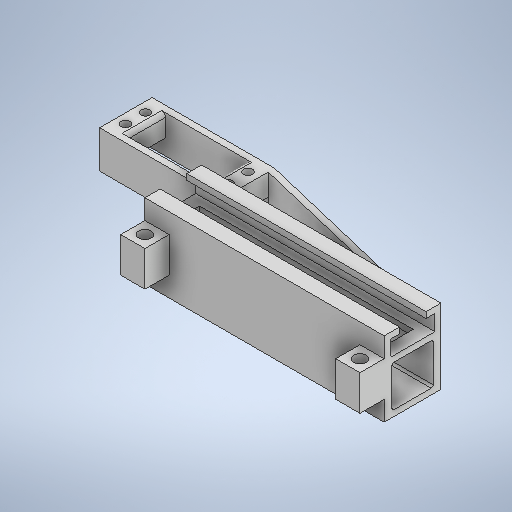
# Autodesk Inventor part: shaftHolder4V1
Saved by Autodesk Inventor 2025.2 (Build 292293000, 293)
## iProperties
Created: 2025-04-03
Part Number: shaftHolder4V1
Material: Generic
Document SubType Name: Modeling
Designer: patrickandersen
Density: 1 g/cm^3
Appearance: Default
Author: patrickandersen
Autodesk Inventor part; units mm, degrees
ref_plane "YZ Plane" through (0, 0, 0) normal (1, 0, 0) x (0, 1, 0)
ref_plane "XZ Plane" through (0, 0, 0) normal (0, 1, 0) x (-1, 0, 0)
ref_plane "XY Plane" through (0, 0, 0) normal (0, 0, 1) x (1, 0, 0)
sketch "Sketch1" plane through (0, 0, 0) normal (0, 1, 0) x (-1, 0, 0)
  line L0 (200.4562, 91.842) -> (79.4562, 91.842)
  line L1 (79.4562, 91.842) -> (79.4562, 63.142)
  line L2 (79.4562, 63.142) -> (200.4562, 63.142)
  line L3 (200.4562, 63.142) -> (200.4562, 91.842)
  point P0 (0, 0)
  dimension "d0" = 121
  dimension "d1" = 28.7
  constraints: 8 end point, 2 parallel, 1 horizontal, 1 perpendicular
  measures "d0" distance of L1.end L2.end
  measures "d1" distance of L0.end L1.end
extrude "Extrusion1" add sketch "Sketch1" along normal blind 26.8
sketch "Sketch2" plane through (-79.4562, 0, 91.842) normal (1, 0, 0) x (0, 0, -1)
  line L0 (4.95, 3) -> (23.75, 3)
  line L1 (24.75, 4) -> (24.75, 22.8)
  line L2 (23.75, 23.8) -> (4.95, 23.8)
  line L3 (3.95, 22.8) -> (3.95, 4)
  line L4 (28.7, 0) -> (28.7, 26.8) projected
  line L5 (0, 0) -> (0, 26.8) projected
  line L6 (0, 26.8) -> (28.7, 26.8) projected
  arc A0 (24.75, 22.8) -> (23.75, 23.8) centre (23.75, 22.8) ccw
  arc A1 (23.75, 3) -> (24.75, 4) centre (23.75, 4) ccw
  arc A2 (3.95, 4) -> (4.95, 3) centre (4.95, 4) ccw
  arc A3 (4.95, 23.8) -> (3.95, 22.8) centre (4.95, 22.8) ccw
  line L7 (0, 0) -> (28.7, 0) projected
  point P0 (91.842, 0)
  point P1 (3.95, 3)
  point P2 (24.75, 23.8)
  point P3 (3.95, 23.8)
  dimension "d4" = 20.8
  dimension "d5" = 20.8
  dimension "d7" = 3.95
  dimension "d8" = 3
  dimension "d9" = 1
  dimension "d137" = 3.95
  dimension "d138" = 3
  constraints: 8 end point, 8 point on circle, 8 tangent, 6 point on line, 4 centre point, 3 equal radius, 2 parallel, 1 horizontal, 1 perpendicular
  measures "d4" distance of point (3.95, 23.8) point (3.95, 3)
  measures "d5" distance of point (24.75, 23.8) point (3.95, 23.8)
  measures "d7" distance between parallel lines of L5 L3
  measures "d8" distance between parallel lines of L6 L2
  measures "d9" radius of A0
  measures "d137" distance between parallel lines of L4 L1
  measures "d138" distance between parallel lines of L7 L0
extrude "Extrusion2" cut sketch "Sketch2" against normal blind 121 contours A2 L3 A3 L2 A0 L1 A1 L0
sketch "Sketch3" plane through (0, 0, 0) normal (0, -1, 0) x (1, 0, 0)
  line L0 (-200.4562, 63.142) -> (-200.4562, 91.842) projected
  line L1 (-200.4562, 91.842) -> (-79.4562, 91.842) projected
  line L2 (-79.4562, 63.142) -> (-200.4562, 63.142) projected
  circle A0 centre (-188.2062, 77.492) radius 9.25
  line L3 (-79.4562, 91.842) -> (-79.4562, 63.142) projected
  point P0 (0, 0)
  dimension "d20" = 14.35
  dimension "d21" = 18.5
  dimension "d287" = 12.25
  constraints: 1 centre point
  measures "d20" distance from line of L1 A0.centre
  measures "d21" diameter of A0
  measures "d287" distance from line of L0 A0.centre
hole "Hole1" at (-188.2062, 0, 77.492) direction (0, 1, 0) diameter 18.5 depth 5
sketch "Sketch4" plane through (0, 26.8, 0) normal (0, 1, 0) x (1, 0, 0)
  line L0 (-85.9562, -84.142) -> (-193.9562, -84.142)
  line L1 (-193.9562, -84.142) -> (-193.9562, -70.642)
  line L2 (-193.9562, -70.642) -> (-85.9562, -70.642)
  line L3 (-85.9562, -70.642) -> (-85.9562, -84.142)
  line L4 (-79.4562, -91.842) -> (-79.4562, -63.142) projected
  line L5 (-200.4562, -63.142) -> (-200.4562, -91.842) projected
  point P0 (0, 0)
  point P1 (-79.4562, -86.142)
  point P2 (-79.4562, -65.142)
  point P3 (-179.4562, -65.142)
  point P4 (-179.4562, -86.142)
  point P5 (-200.4562, -91.842)
  point P6 (-79.4562, -87.892)
  dimension "d30" = 6.5
  dimension "d31" = 6.5
  dimension "d32" = 13.5
  dimension "d41" = 3.75
  constraints: 8 end point, 2 parallel, 1 horizontal, 1 perpendicular, 1 other
  measures "d30" distance between parallel lines of L4 L3
  measures "d32" distance between parallel lines of L0 L2
  measures "d41" distance from line of point (-79.456, -87.892) L0
extrude "Extrusion3" cut sketch "Sketch4" against normal blind 5
sketch "Sketch5" plane through (0, 26.8, 0) normal (0, 1, 0) x (1, 0, 0)
  line L0 (-79.4562, -91.842) -> (-79.4562, -63.142) projected
  line L1 (-200.4562, -63.142) -> (-200.4562, -91.842) projected
  line L2 (-79.4562, -91.842) -> (-200.4562, -91.842)
  line L3 (-200.4562, -91.842) -> (-200.4562, -88.442)
  line L4 (-200.4562, -88.442) -> (-79.4562, -88.442)
  line L5 (-79.4562, -88.442) -> (-79.4562, -91.842)
  line L6 (-79.4562, -63.142) -> (-200.4562, -63.142)
  line L7 (-200.4562, -63.142) -> (-200.4562, -66.142)
  line L8 (-200.4562, -66.142) -> (-79.4562, -66.142)
  line L9 (-79.4562, -66.142) -> (-79.4562, -63.142)
  line L10 (-79.4562, -63.142) -> (-200.4562, -63.142) projected
  line L11 (-79.4562, -87.892) -> (-79.4562, -87.642)
  line L12 (-79.4562, -87.642) -> (-79.4562, -81.492)
  point P0 (0, 0)
  point P1 (-79.4562, -66.142)
  dimension "d38" = 3.4
  dimension "d39" = 3
  dimension "d40" = 0
  dimension "d42" = 22.3
  dimension "d288" = 0.25
  dimension "d289" = 6.15
  constraints: 20 end point, 5 point on line, 4 parallel, 2 horizontal, 2 perpendicular
  measures "d38" distance between parallel lines of L2 L4
  measures "d39" distance between parallel lines of L6 L8
  measures "d40" distance between parallel lines of L10 L6
  measures "d42" distance between parallel lines of L8 L4
  measures "d288" distance of L11.start L11.end
  measures "d289" distance of L11.end L12.end
extrude "Extrusion4" add sketch "Sketch5" along normal blind 8 contours L2 L1 L4 L0 | L1 L6 L0 L8
sketch "Sketch6" plane through (0, 34.8, 0) normal (0, 1, 0) x (1, 0, 0)
  line L0 (-200.4562, -91.842) -> (-79.4562, -91.842) projected
  line L1 (-200.4562, -66.142) -> (-200.4562, -88.442) projected
  line L2 (-79.4562, -91.842) -> (-200.4562, -91.842)
  line L3 (-200.4562, -91.842) -> (-200.4562, -84.142)
  line L4 (-200.4562, -84.142) -> (-79.4562, -84.142)
  line L5 (-79.4562, -84.142) -> (-79.4562, -91.842)
  line L6 (-79.4562, -63.142) -> (-200.4562, -63.142) projected
  line L7 (-79.4562, -63.142) -> (-200.4562, -63.142)
  line L8 (-200.4562, -63.142) -> (-200.4562, -70.642)
  line L9 (-200.4562, -70.642) -> (-79.4562, -70.642)
  line L10 (-79.4562, -70.642) -> (-79.4562, -63.142)
  line L11 (-85.9562, -84.142) -> (-193.9562, -84.142) projected
  line L12 (-193.9562, -70.642) -> (-85.9562, -70.642) projected
  point P0 (0, 0)
  point P1 (-200.4562, -91.842)
  dimension "d45" = 0
  dimension "d46" = 0
  constraints: 16 end point, 4 parallel, 2 horizontal, 2 perpendicular, 2 point on line
  measures "d45" distance between parallel lines of L11 L4
  measures "d46" distance between parallel lines of L12 L9
extrude "Extrusion5" add sketch "Sketch6" along normal blind 3
sketch "Sketch11" plane through (-79.4562, 0, 63.142) normal (0, 0, -1) x (-1, 0, 0)
  line L0 (172.6, 9.3) -> (0, 9.3)
  line L1 (0, 9.3) -> (0, 28.3)
  line L2 (0, 28.3) -> (172.6, 28.3)
  line L3 (172.6, 28.3) -> (172.6, 9.3)
  line L4 (0, 37.8) -> (121, 37.8) projected
  line L5 (0, 0) -> (0, 37.8) projected
  line L6 (0, 0) -> (121, 0) projected
  line L7 (0, 28.3) -> (0, 49.8)
  line L8 (0, 34.8) -> (121, 34.8) projected
  line L9 (121, 0) -> (121, 37.8) projected
  point P0 (-79.4562, 0)
  point P1 (0, 3)
  dimension "d97" = 0
  dimension "d105" = 12
  dimension "d110" = 9.5
  dimension "d111" = 21.5
  dimension "d113" = 19
  dimension "d114" = 9.3
  dimension "d174" = 51.6
  constraints: 10 end point, 2 parallel, 1 horizontal, 1 perpendicular, 1 vertical
  measures "d97" distance between parallel lines of L5 L1
  measures "d105" distance from line of L4 L7.end
  measures "d110" distance between parallel lines of L2 L4
  measures "d111" distance from line of L7.end L2
  measures "d113" distance of L2.end L0.start
  measures "d114" distance between parallel lines of L6 L0
  measures "d174" distance between parallel lines of L9 L3
extrude "Extrusion9" add sketch "Sketch11" along normal blind 26.5 contours L0 L9 L2 L3 | L0 L1 L2 L9
sketch "Sketch12" plane through (-252.0562, 28.3, 63.142) normal (0, 1, 0) x (1, 0, 0)
  line L0 (51.6, 3.25) -> (10.1, 3.25)
  line L1 (10.1, 3.25) -> (10.1, 23.25)
  line L2 (10.1, 23.25) -> (51.6, 23.25)
  line L3 (51.6, 23.25) -> (51.6, 3.25)
  line L4 (0, 0) -> (51.6, 0) projected
  line L5 (0, 26.5) -> (172.6, 26.5) projected
  line L6 (0, 0) -> (0, 26.5) projected
  line L7 (51.6, 0) -> (51.6, -7.5) projected
  line L8 (172.6, 0) -> (51.6, 0) projected
  line L9 (172.6, 0) -> (172.6, 26.5) projected
  point P0 (252.0562, 63.142)
  point P1 (49.2771, 26.5)
  point P2 (51.6, -3.75)
  point P3 (82, 26.5)
  dimension "d120" = 41.5
  dimension "d121" = 20
  dimension "d122" = 3.25
  dimension "d123" = 3.25
  dimension "d127" = 0
  dimension "d128" = 10.1
  constraints: 8 end point, 2 parallel, 1 horizontal, 1 midpoint, 1 perpendicular
  measures "d120" distance of L0.start L0.end
  measures "d121" distance of L0.end L1.end
  measures "d122" distance between parallel lines of L4 L0
  measures "d123" distance between parallel lines of L5 L2
  measures "d127" distance from line of point (51.6, -3.75) L3
  measures "d128" distance between parallel lines of L6 L1
extrude "Extrusion10" cut sketch "Sketch12" against normal blind 26.5 contours L0 L1 L2 L3
sketch "Sketch14" plane through (-252.0562, 28.3, 63.142) normal (0, 1, 0) x (1, 0, 0)
  circle A0 centre (4.85, 8.25) radius 2.25
  circle A1 centre (4.85, 18.25) radius 2.25
  circle A2 centre (56.85, 8.25) radius 2.25
  circle A3 centre (56.85, 18.25) radius 2.25
  line L0 (10.1, 3.25) -> (10.1, 23.25) projected
  line L1 (51.6, 23.25) -> (51.6, 3.25) projected
  line L2 (0, 0) -> (0, 26.5) projected
  line L3 (51.6, 3.25) -> (10.1, 3.25) projected
  point P0 (252.0562, 63.142)
  dimension "d141" = 4.5
  dimension "d142" = 4.5
  dimension "d143" = 4.5
  dimension "d144" = 4.5
  dimension "d145" = 5.25
  dimension "d146" = 5.25
  dimension "d148" = 4.85
  dimension "d149" = 5.25
  dimension "d150" = 10
  dimension "d151" = 5
  dimension "d153" = 5.25
  dimension "d154" = 10
  dimension "d155" = 5
  constraints: 4 centre point
  measures "d141" diameter of A0
  measures "d142" diameter of A1
  measures "d143" diameter of A2
  measures "d144" diameter of A3
  measures "d145" distance from line of L0 A0.centre
  measures "d146" distance from line of L1 A2.centre
  measures "d148" distance from line of L2 A0.centre
  measures "d149" distance from line of L0 A1.centre
  measures "d150" distance of A1.centre A0.centre
  measures "d151" distance from line of L3 A0.centre
  measures "d153" distance from line of L1 A3.centre
  measures "d154" distance of A3.centre A2.centre
  measures "d155" distance from line of L3 A2.centre
sketch "Sketch15" plane through (-252.0562, 9.3, 63.142) normal (-1, 0, 0) x (0, 0, 1)
  line L0 (-23.25, 0) -> (-3.25, 0)
  line L1 (-3.25, 0) -> (-3.25, 14)
  line L2 (-3.25, 14) -> (-23.25, 14)
  line L3 (-23.25, 14) -> (-23.25, 0)
  line L4 (-26.5, 0) -> (-26.5, 19) projected
  line L5 (0, 0) -> (0, 19) projected
  line L6 (0, 0) -> (-26.5, 0) projected
  line L7 (0, 19) -> (-26.5, 19) projected
  point P0 (-63.142, -9.3)
  dimension "d156" = 3.25
  dimension "d157" = 3.25
  dimension "d158" = 0
  dimension "d159" = 5
  constraints: 8 end point, 2 parallel, 1 horizontal, 1 perpendicular
  measures "d156" distance between parallel lines of L4 L3
  measures "d157" distance between parallel lines of L5 L1
  measures "d158" distance between parallel lines of L6 L0
  measures "d159" distance between parallel lines of L7 L2
extrude "Extrusion11" cut sketch "Sketch15" against normal blind 62 contours L3 L2 L1 L0
hole "Hole3" at (-195.2062, 28.3, 44.892) at (-195.2062, 28.3, 54.892) at (-247.2062, 28.3, 54.892) at (-247.2062, 28.3, 44.892) direction (0, -1, 0) diameter 4.5 depth 6
sketch "Sketch19" plane through (-200.4562, 23.3, 39.892) normal (0, -1, 0) x (1, 0, 0)
  circle A0 centre (5.25, 5) radius 2.25 projected
  line L0 (3.1571, 1.375) -> (1.0642, 5)
  line L1 (1.0642, 5) -> (3.1571, 8.625)
  line L2 (3.1571, 8.625) -> (7.3429, 8.625)
  line L3 (7.3429, 8.625) -> (9.4358, 5)
  line L4 (9.4358, 5) -> (7.3429, 1.375)
  line L5 (7.3429, 1.375) -> (3.1571, 1.375)
  circle A1 centre (5.25, 15) radius 2.25 projected
  line L6 (3.1571, 11.375) -> (1.0642, 15)
  line L7 (1.0642, 15) -> (3.1571, 18.625)
  line L8 (3.1571, 18.625) -> (7.3429, 18.625)
  line L9 (7.3429, 18.625) -> (9.4358, 15)
  line L10 (9.4358, 15) -> (7.3429, 11.375)
  line L11 (7.3429, 11.375) -> (3.1571, 11.375)
  circle A2 centre (-46.75, 5) radius 2.25 projected
  line L12 (-50.9358, 5) -> (-48.8429, 8.625)
  line L13 (-48.8429, 8.625) -> (-44.6571, 8.625)
  line L14 (-44.6571, 8.625) -> (-42.5642, 5)
  line L15 (-42.5642, 5) -> (-44.6571, 1.375)
  line L16 (-44.6571, 1.375) -> (-48.8429, 1.375)
  line L17 (-48.8429, 1.375) -> (-50.9358, 5)
  circle A3 centre (-46.75, 15) radius 2.25 projected
  line L18 (-50.9358, 15) -> (-48.8429, 18.625)
  line L19 (-48.8429, 18.625) -> (-44.6571, 18.625)
  line L20 (-44.6571, 18.625) -> (-42.5642, 15)
  line L21 (-42.5642, 15) -> (-44.6571, 11.375)
  line L22 (-44.6571, 11.375) -> (-48.8429, 11.375)
  line L23 (-48.8429, 11.375) -> (-50.9358, 15)
  line L24 (0, 0) -> (0, 20) projected
  line L25 (0, 0) -> (0, 20)
  line L26 (10.4, 0) -> (0, 0)
  line L27 (0, 0) -> (0, 20)
  line L28 (0, 20) -> (10.4, 20)
  line L29 (10.4, 20) -> (10.4, 0)
  line L30 (-51.6, 0) -> (-51.6, 20) projected
  line L31 (-41.5, 0) -> (-51.6, 0)
  line L32 (-51.6, 0) -> (-51.6, 20)
  line L33 (-51.6, 20) -> (-41.5, 20)
  line L34 (-41.5, 20) -> (-41.5, 0)
  point P0 (200.4562, -39.892)
  point P1 (5.25, 15)
  point P2 (-51.6, 0)
  dimension "d191" = 7.25
  dimension "d194" = 7.25
  dimension "d197" = 0
  dimension "d198" = 0
  dimension "d199" = 7.25
  dimension "d200" = 7.25
  constraints: 66 end point, 4 coincident, 4 parallel, 2 horizontal, 2 perpendicular, 1 vertical, 52 other
  measures "d191" distance between parallel lines of L4 L1
  measures "d194" distance between parallel lines of L10 L7
  measures "d197" vertical distance of L6.end point (5.25, 15)
  measures "d198" vertical distance of L0.end point (5.25, 5)
  measures "d199" distance between parallel lines of L22 L19
  measures "d200" distance between parallel lines of L16 L13
extrude "Extrusion14" add sketch "Sketch19" along normal blind 6 contours L24 L28 L29 L26 | L30 L33 L34 L31
fillet "Fillet8" radius 2 2 edges at (-200.4562, 28.3, 49.892) (-241.9562, 28.3, 49.892)
sketch "Sketch25" plane through (-200.4562, 0, 91.842) normal (0, 0, 1) x (1, 0, 0)
  line L0 (0, 27.8) -> (12.25, 27.8)
  line L1 (12.25, 27.8) -> (12.25, 10)
  line L2 (12.25, 10) -> (0, 10)
  line L3 (0, 10) -> (0, 27.8)
  line L4 (0, 0) -> (0, 37.8) projected
  line L5 (0, 37.8) -> (121, 37.8) projected
  line L6 (0, 0) -> (121, 0) projected
  line L7 (108.75, 27.8) -> (121, 27.8)
  line L8 (121, 27.8) -> (121, 10)
  line L9 (121, 10) -> (108.75, 10)
  line L10 (108.75, 10) -> (108.75, 27.8)
  line L11 (121, 0) -> (121, 37.8) projected
  point P0 (200.4562, 0)
  dimension "d250" = 0
  dimension "d251" = 37.8
  dimension "d252" = 10
  dimension "d253" = 10
  dimension "d254" = 0
  dimension "d255" = 10
  dimension "d256" = 10
  dimension "d257" = 12.25
  dimension "d258" = 12.25
  constraints: 16 end point, 4 parallel, 2 horizontal, 2 perpendicular
  measures "d250" distance between parallel lines of L4 L3
  measures "d251" distance of L4.start L4.end
  measures "d252" distance between parallel lines of L5 L0
  measures "d253" distance between parallel lines of L6 L2
  measures "d254" distance between parallel lines of L11 L8
  measures "d255" distance between parallel lines of L5 L7
  measures "d256" distance between parallel lines of L6 L9
  measures "d257" distance of L0.start L0.end
  measures "d258" distance of L7.start L7.end
extrude "Extrusion18" add sketch "Sketch25" along normal blind 12.25 contours L0 L1 L2 L3
extrude "Extrusion19" add sketch "Sketch25" along normal blind 12.25 contours L8 L9 L10 L7
sketch "Sketch26" plane through (-200.4562, 27.8, 91.842) normal (0, 1, 0) x (1, 0, 0)
  circle A0 centre (6.125, -6.125) radius 3.125
  line L0 (12.25, 0) -> (12.25, -12.25) projected
  line L1 (12.25, -12.25) -> (0, -12.25) projected
  circle A1 centre (114.875, -6.125) radius 3.125
  line L2 (121, 0) -> (121, -12.25) projected
  line L3 (121, -12.25) -> (108.75, -12.25) projected
  point P0 (200.4562, 91.842)
  dimension "d263" = 6.25
  dimension "d266" = 6.125
  dimension "d267" = 6.125
  dimension "d268" = 6.25
  dimension "d269" = 6.125
  dimension "d270" = 6.125
  constraints: 2 centre point
  measures "d263" diameter of A0
  measures "d266" distance from line of L0 A0.centre
  measures "d267" distance from line of L1 A0.centre
  measures "d268" diameter of A1
  measures "d269" distance from line of L2 A1.centre
  measures "d270" distance from line of L3 A1.centre
hole "Hole5" at (-194.3312, 27.8, 97.967) at (-85.5812, 27.8, 97.967) direction (0, -1, 0) diameter 6.25 depth 20
sketch "Sketch28" plane through (-252.0562, 28.3, 63.142) normal (0, 1, 0) x (1, 0, 0)
  line L0 (172.6, 0) -> (172.6, 26.5) projected
  line L1 (62, 3.25) -> (62, 23.25) projected
  line L2 (0, 3.25) -> (62, 3.25) projected
  line L3 (172.6, 0) -> (172.6, 26.5)
  line L4 (172.6, 26.5) -> (172.6, 0)
  line L5 (172.6, 26.5) -> (62, 26.5)
  line L6 (0, 26.5) -> (172.6, 26.5) projected
  line L7 (62, 26.5) -> (172.6, 0)
  line L8 (62, 23.25) -> (158.9481, 0)
  line L9 (172.6, 0) -> (51.6, 0) projected
  line L10 (62, 3.25) -> (145.3962, 3.25)
  point P0 (252.0562, 63.142)
  constraints: 12 end point, 3 point on line, 2 collinear, 1 horizontal
extrude "Extrusion20" cut sketch "Sketch28" against normal blind 30
fillet "Fillet12" radius 1 1 edges at (-190.0562, 18.8, 36.642)
fillet "Fillet13" radius 0.5 1 edges at (-139.9562, 34.8, 88.442)
fillet "Fillet14" radius 0.5 1 edges at (-139.9562, 26.8, 88.442)
body "Solid1"
